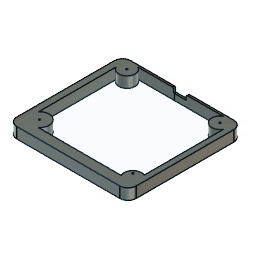
case (Autodesk Fusion 360 design; units mm, degrees)
description: KiCad electronic assembly
part number: case 1
Autodesk Fusion 360 part; units mm, degrees
(part 1 of 2)
sketch "Sketch1" plane through (0, 0, -0.05) normal (0, 0, -1) x (1, 0, 0)
  arc A0 (115.9024, 71.5818) -> (120.6818, 66.8024) centre (120.9, 71.8) ccw
  line L0 (120.6818, 66.8024) -> (120.9, 66.8)
  line L1 (120.9, 66.8) -> (209.95, 66.8)
  line L2 (209.95, 66.8) -> (210.1682, 66.8024)
  arc A1 (210.1682, 66.8024) -> (214.9476, 71.5818) centre (209.95, 71.8) ccw
  line L3 (214.9476, 71.5818) -> (214.95, 71.8)
  line L4 (214.95, 71.8) -> (214.95, 155.9)
  line L5 (214.95, 155.9) -> (214.9476, 156.1182)
  arc A2 (214.9476, 156.1182) -> (210.1682, 160.8976) centre (209.95, 155.9) ccw
  line L6 (210.1682, 160.8976) -> (209.95, 160.9)
  line L7 (209.95, 160.9) -> (120.9, 160.9)
  line L8 (120.9, 160.9) -> (120.6818, 160.8976)
  arc A3 (120.6818, 160.8976) -> (115.9024, 156.1182) centre (120.9, 155.9) ccw
  line L9 (115.9024, 156.1182) -> (115.9, 155.9)
  line L10 (115.9, 155.9) -> (115.9, 71.8)
  line L11 (115.9, 71.8) -> (115.9024, 71.5818)
  circle A4 centre (122.55, 154.05) radius 2.2
  circle A5 centre (208.4, 153.95) radius 2.2
  arc A6 (188.315, 150.698) -> (188.417, 150.8) centre (188.315, 150.8) ccw
  line L12 (188.315, 150.698) -> (187.415, 150.698)
  arc A7 (187.313, 150.8) -> (187.415, 150.698) centre (187.415, 150.8) ccw
  line L13 (187.313, 150.8) -> (187.313, 152.3)
  arc A8 (187.415, 152.402) -> (187.313, 152.3) centre (187.415, 152.3) ccw
  line L14 (187.415, 152.402) -> (188.315, 152.402)
  arc A9 (188.417, 152.3) -> (188.315, 152.402) centre (188.315, 152.3) ccw
  line L15 (188.417, 152.3) -> (188.417, 150.8)
  arc A10 (189.585, 150.698) -> (189.687, 150.8) centre (189.585, 150.8) ccw
  line L16 (189.585, 150.698) -> (188.685, 150.698)
  arc A11 (188.583, 150.8) -> (188.685, 150.698) centre (188.685, 150.8) ccw
  line L17 (188.583, 150.8) -> (188.583, 152.3)
  arc A12 (188.685, 152.402) -> (188.583, 152.3) centre (188.685, 152.3) ccw
  line L18 (188.685, 152.402) -> (189.585, 152.402)
  arc A13 (189.687, 152.3) -> (189.585, 152.402) centre (189.585, 152.3) ccw
  line L19 (189.687, 152.3) -> (189.687, 150.8)
  arc A14 (190.855, 150.698) -> (190.957, 150.8) centre (190.855, 150.8) ccw
  line L20 (190.855, 150.698) -> (189.955, 150.698)
  arc A15 (189.853, 150.8) -> (189.955, 150.698) centre (189.955, 150.8) ccw
  line L21 (189.853, 150.8) -> (189.853, 152.3)
  arc A16 (189.955, 152.402) -> (189.853, 152.3) centre (189.955, 152.3) ccw
  line L22 (189.955, 152.402) -> (190.855, 152.402)
  arc A17 (190.957, 152.3) -> (190.855, 152.402) centre (190.855, 152.3) ccw
  line L23 (190.957, 152.3) -> (190.957, 150.8)
  arc A18 (192.125, 150.698) -> (192.227, 150.8) centre (192.125, 150.8) ccw
  line L24 (192.125, 150.698) -> (191.225, 150.698)
  arc A19 (191.123, 150.8) -> (191.225, 150.698) centre (191.225, 150.8) ccw
  line L25 (191.123, 150.8) -> (191.123, 152.3)
  arc A20 (191.225, 152.402) -> (191.123, 152.3) centre (191.225, 152.3) ccw
  line L26 (191.225, 152.402) -> (192.125, 152.402)
  arc A21 (192.227, 152.3) -> (192.125, 152.402) centre (192.125, 152.3) ccw
  line L27 (192.227, 152.3) -> (192.227, 150.8)
  arc A22 (193.395, 150.698) -> (193.497, 150.8) centre (193.395, 150.8) ccw
  line L28 (193.395, 150.698) -> (192.495, 150.698)
  arc A23 (192.393, 150.8) -> (192.495, 150.698) centre (192.495, 150.8) ccw
  line L29 (192.393, 150.8) -> (192.393, 152.3)
  arc A24 (192.495, 152.402) -> (192.393, 152.3) centre (192.495, 152.3) ccw
  line L30 (192.495, 152.402) -> (193.395, 152.402)
  arc A25 (193.497, 152.3) -> (193.395, 152.402) centre (193.395, 152.3) ccw
  line L31 (193.497, 152.3) -> (193.497, 150.8)
  arc A26 (194.665, 150.698) -> (194.767, 150.8) centre (194.665, 150.8) ccw
  line L32 (194.665, 150.698) -> (193.765, 150.698)
  arc A27 (193.663, 150.8) -> (193.765, 150.698) centre (193.765, 150.8) ccw
  line L33 (193.663, 150.8) -> (193.663, 152.3)
  arc A28 (193.765, 152.402) -> (193.663, 152.3) centre (193.765, 152.3) ccw
  line L34 (193.765, 152.402) -> (194.665, 152.402)
  arc A29 (194.767, 152.3) -> (194.665, 152.402) centre (194.665, 152.3) ccw
  line L35 (194.767, 152.3) -> (194.767, 150.8)
  arc A30 (195.935, 150.698) -> (196.037, 150.8) centre (195.935, 150.8) ccw
  line L36 (195.935, 150.698) -> (195.035, 150.698)
  arc A31 (194.933, 150.8) -> (195.035, 150.698) centre (195.035, 150.8) ccw
  line L37 (194.933, 150.8) -> (194.933, 152.3)
  arc A32 (195.035, 152.402) -> (194.933, 152.3) centre (195.035, 152.3) ccw
  line L38 (195.035, 152.402) -> (195.935, 152.402)
  arc A33 (196.037, 152.3) -> (195.935, 152.402) centre (195.935, 152.3) ccw
  line L39 (196.037, 152.3) -> (196.037, 150.8)
  arc A34 (197.205, 150.698) -> (197.307, 150.8) centre (197.205, 150.8) ccw
  line L40 (197.205, 150.698) -> (196.305, 150.698)
  arc A35 (196.203, 150.8) -> (196.305, 150.698) centre (196.305, 150.8) ccw
  line L41 (196.203, 150.8) -> (196.203, 152.3)
  arc A36 (196.305, 152.402) -> (196.203, 152.3) centre (196.305, 152.3) ccw
  line L42 (196.305, 152.402) -> (197.205, 152.402)
  arc A37 (197.307, 152.3) -> (197.205, 152.402) centre (197.205, 152.3) ccw
  line L43 (197.307, 152.3) -> (197.307, 150.8)
  arc A38 (198.475, 150.698) -> (198.577, 150.8) centre (198.475, 150.8) ccw
  line L44 (198.475, 150.698) -> (197.575, 150.698)
  arc A39 (197.473, 150.8) -> (197.575, 150.698) centre (197.575, 150.8) ccw
  line L45 (197.473, 150.8) -> (197.473, 152.3)
  arc A40 (197.575, 152.402) -> (197.473, 152.3) centre (197.575, 152.3) ccw
  line L46 (197.575, 152.402) -> (198.475, 152.402)
  arc A41 (198.577, 152.3) -> (198.475, 152.402) centre (198.475, 152.3) ccw
  line L47 (198.577, 152.3) -> (198.577, 150.8)
  arc A42 (199.745, 150.698) -> (199.847, 150.8) centre (199.745, 150.8) ccw
  line L48 (199.745, 150.698) -> (198.845, 150.698)
  arc A43 (198.743, 150.8) -> (198.845, 150.698) centre (198.845, 150.8) ccw
  line L49 (198.743, 150.8) -> (198.743, 152.3)
  arc A44 (198.845, 152.402) -> (198.743, 152.3) centre (198.845, 152.3) ccw
  line L50 (198.845, 152.402) -> (199.745, 152.402)
  arc A45 (199.847, 152.3) -> (199.745, 152.402) centre (199.745, 152.3) ccw
  line L51 (199.847, 152.3) -> (199.847, 150.8)
  arc A46 (201.015, 150.698) -> (201.117, 150.8) centre (201.015, 150.8) ccw
  line L52 (201.015, 150.698) -> (200.115, 150.698)
  arc A47 (200.013, 150.8) -> (200.115, 150.698) centre (200.115, 150.8) ccw
  line L53 (200.013, 150.8) -> (200.013, 152.3)
  arc A48 (200.115, 152.402) -> (200.013, 152.3) centre (200.115, 152.3) ccw
  line L54 (200.115, 152.402) -> (201.015, 152.402)
  arc A49 (201.117, 152.3) -> (201.015, 152.402) centre (201.015, 152.3) ccw
  line L55 (201.117, 152.3) -> (201.117, 150.8)
  arc A50 (202.285, 150.698) -> (202.387, 150.8) centre (202.285, 150.8) ccw
  line L56 (202.285, 150.698) -> (201.385, 150.698)
  arc A51 (201.283, 150.8) -> (201.385, 150.698) centre (201.385, 150.8) ccw
  line L57 (201.283, 150.8) -> (201.283, 152.3)
  arc A52 (201.385, 152.402) -> (201.283, 152.3) centre (201.385, 152.3) ccw
  line L58 (201.385, 152.402) -> (202.285, 152.402)
  arc A53 (202.387, 152.3) -> (202.285, 152.402) centre (202.285, 152.3) ccw
  line L59 (202.387, 152.3) -> (202.387, 150.8)
  arc A54 (183.55, 150.523) -> (183.652, 150.625) centre (183.55, 150.625) ccw
  line L60 (183.55, 150.523) -> (181.4, 150.523)
  arc A55 (181.298, 150.625) -> (181.4, 150.523) centre (181.4, 150.625) ccw
  line L61 (181.298, 150.625) -> (181.298, 151.575)
  arc A56 (181.4, 151.677) -> (181.298, 151.575) centre (181.4, 151.575) ccw
  line L62 (181.4, 151.677) -> (183.55, 151.677)
  arc A57 (183.652, 151.575) -> (183.55, 151.677) centre (183.55, 151.575) ccw
  line L63 (183.652, 151.575) -> (183.652, 150.625)
  arc A58 (186.85, 149.748) -> (186.952, 149.85) centre (186.85, 149.85) ccw
  line L64 (186.85, 149.748) -> (185.35, 149.748)
  arc A59 (185.248, 149.85) -> (185.35, 149.748) centre (185.35, 149.85) ccw
  line L65 (185.248, 149.85) -> (185.248, 150.75)
  arc A60 (185.35, 150.852) -> (185.248, 150.75) centre (185.35, 150.75) ccw
  line L66 (185.35, 150.852) -> (186.85, 150.852)
  arc A61 (186.952, 150.75) -> (186.85, 150.852) centre (186.85, 150.75) ccw
  line L67 (186.952, 150.75) -> (186.952, 149.85)
  arc A62 (204.35, 149.748) -> (204.452, 149.85) centre (204.35, 149.85) ccw
  line L68 (204.35, 149.748) -> (202.85, 149.748)
  arc A63 (202.748, 149.85) -> (202.85, 149.748) centre (202.85, 149.85) ccw
  line L69 (202.748, 149.85) -> (202.748, 150.75)
  arc A64 (202.85, 150.852) -> (202.748, 150.75) centre (202.85, 150.75) ccw
  line L70 (202.85, 150.852) -> (204.35, 150.852)
  arc A65 (204.452, 150.75) -> (204.35, 150.852) centre (204.35, 150.75) ccw
  line L71 (204.452, 150.75) -> (204.452, 149.85)
  arc A66 (177.75, 147.073) -> (177.852, 147.175) centre (177.75, 147.175) ccw
  line L72 (177.75, 147.073) -> (175.6, 147.073)
  arc A67 (175.498, 147.175) -> (175.6, 147.073) centre (175.6, 147.175) ccw
  line L73 (175.498, 147.175) -> (175.498, 150.425)
  arc A68 (175.6, 150.527) -> (175.498, 150.425) centre (175.6, 150.425) ccw
  line L74 (175.6, 150.527) -> (177.75, 150.527)
  arc A69 (177.852, 150.425) -> (177.75, 150.527) centre (177.75, 150.425) ccw
  line L75 (177.852, 150.425) -> (177.852, 147.175)
  arc A70 (186.85, 148.478) -> (186.952, 148.58) centre (186.85, 148.58) ccw
  line L76 (186.85, 148.478) -> (185.35, 148.478)
  arc A71 (185.248, 148.58) -> (185.35, 148.478) centre (185.35, 148.58) ccw
  line L77 (185.248, 148.58) -> (185.248, 149.48)
  arc A72 (185.35, 149.582) -> (185.248, 149.48) centre (185.35, 149.48) ccw
  line L78 (185.35, 149.582) -> (186.85, 149.582)
  arc A73 (186.952, 149.48) -> (186.85, 149.582) centre (186.85, 149.48) ccw
  line L79 (186.952, 149.48) -> (186.952, 148.58)
  arc A74 (204.35, 148.478) -> (204.452, 148.58) centre (204.35, 148.58) ccw
  line L80 (204.35, 148.478) -> (202.85, 148.478)
  arc A75 (202.748, 148.58) -> (202.85, 148.478) centre (202.85, 148.58) ccw
  line L81 (202.748, 148.58) -> (202.748, 149.48)
  arc A76 (202.85, 149.582) -> (202.748, 149.48) centre (202.85, 149.48) ccw
  line L82 (202.85, 149.582) -> (204.35, 149.582)
  arc A77 (204.452, 149.48) -> (204.35, 149.582) centre (204.35, 149.48) ccw
  line L83 (204.452, 149.48) -> (204.452, 148.58)
  arc A78 (183.55, 148.223) -> (183.652, 148.325) centre (183.55, 148.325) ccw
  line L84 (183.55, 148.223) -> (181.4, 148.223)
  arc A79 (181.298, 148.325) -> (181.4, 148.223) centre (181.4, 148.325) ccw
  line L85 (181.298, 148.325) -> (181.298, 149.275)
  arc A80 (181.4, 149.377) -> (181.298, 149.275) centre (181.4, 149.275) ccw
  line L86 (181.4, 149.377) -> (183.55, 149.377)
  arc A81 (183.652, 149.275) -> (183.55, 149.377) centre (183.55, 149.275) ccw
  line L87 (183.652, 149.275) -> (183.652, 148.325)
  arc A82 (186.85, 147.208) -> (186.952, 147.31) centre (186.85, 147.31) ccw
  line L88 (186.85, 147.208) -> (185.35, 147.208)
  arc A83 (185.248, 147.31) -> (185.35, 147.208) centre (185.35, 147.31) ccw
  line L89 (185.248, 147.31) -> (185.248, 148.21)
  arc A84 (185.35, 148.312) -> (185.248, 148.21) centre (185.35, 148.21) ccw
  line L90 (185.35, 148.312) -> (186.85, 148.312)
  arc A85 (186.952, 148.21) -> (186.85, 148.312) centre (186.85, 148.21) ccw
  line L91 (186.952, 148.21) -> (186.952, 147.31)
  arc A86 (204.35, 147.208) -> (204.452, 147.31) centre (204.35, 147.31) ccw
  line L92 (204.35, 147.208) -> (202.85, 147.208)
  arc A87 (202.748, 147.31) -> (202.85, 147.208) centre (202.85, 147.31) ccw
  line L93 (202.748, 147.31) -> (202.748, 148.21)
  arc A88 (202.85, 148.312) -> (202.748, 148.21) centre (202.85, 148.21) ccw
  line L94 (202.85, 148.312) -> (204.35, 148.312)
  arc A89 (204.452, 148.21) -> (204.35, 148.312) centre (204.35, 148.21) ccw
  line L95 (204.452, 148.21) -> (204.452, 147.31)
  arc A90 (183.55, 145.923) -> (183.652, 146.025) centre (183.55, 146.025) ccw
  line L96 (183.55, 145.923) -> (181.4, 145.923)
  arc A91 (181.298, 146.025) -> (181.4, 145.923) centre (181.4, 146.025) ccw
  line L97 (181.298, 146.025) -> (181.298, 146.975)
  arc A92 (181.4, 147.077) -> (181.298, 146.975) centre (181.4, 146.975) ccw
  line L98 (181.4, 147.077) -> (183.55, 147.077)
  arc A93 (183.652, 146.975) -> (183.55, 147.077) centre (183.55, 146.975) ccw
  line L99 (183.652, 146.975) -> (183.652, 146.025)
  arc A94 (186.85, 145.938) -> (186.952, 146.04) centre (186.85, 146.04) ccw
  line L100 (186.85, 145.938) -> (185.35, 145.938)
  arc A95 (185.248, 146.04) -> (185.35, 145.938) centre (185.35, 146.04) ccw
  line L101 (185.248, 146.04) -> (185.248, 146.94)
  arc A96 (185.35, 147.042) -> (185.248, 146.94) centre (185.35, 146.94) ccw
  line L102 (185.35, 147.042) -> (186.85, 147.042)
  arc A97 (186.952, 146.94) -> (186.85, 147.042) centre (186.85, 146.94) ccw
  line L103 (186.952, 146.94) -> (186.952, 146.04)
  arc A98 (204.35, 145.938) -> (204.452, 146.04) centre (204.35, 146.04) ccw
  line L104 (204.35, 145.938) -> (202.85, 145.938)
  arc A99 (202.748, 146.04) -> (202.85, 145.938) centre (202.85, 146.04) ccw
  line L105 (202.748, 146.04) -> (202.748, 146.94)
  arc A100 (202.85, 147.042) -> (202.748, 146.94) centre (202.85, 146.94) ccw
  line L106 (202.85, 147.042) -> (204.35, 147.042)
  arc A101 (204.452, 146.94) -> (204.35, 147.042) centre (204.35, 146.94) ccw
  line L107 (204.452, 146.94) -> (204.452, 146.04)
  arc A102 (186.85, 144.668) -> (186.952, 144.77) centre (186.85, 144.77) ccw
  line L108 (186.85, 144.668) -> (185.35, 144.668)
  arc A103 (185.248, 144.77) -> (185.35, 144.668) centre (185.35, 144.77) ccw
  line L109 (185.248, 144.77) -> (185.248, 145.67)
  arc A104 (185.35, 145.772) -> (185.248, 145.67) centre (185.35, 145.67) ccw
  line L110 (185.35, 145.772) -> (186.85, 145.772)
  arc A105 (186.952, 145.67) -> (186.85, 145.772) centre (186.85, 145.67) ccw
  line L111 (186.952, 145.67) -> (186.952, 144.77)
  arc A106 (204.35, 144.668) -> (204.452, 144.77) centre (204.35, 144.77) ccw
  line L112 (204.35, 144.668) -> (202.85, 144.668)
  arc A107 (202.748, 144.77) -> (202.85, 144.668) centre (202.85, 144.77) ccw
  line L113 (202.748, 144.77) -> (202.748, 145.67)
  arc A108 (202.85, 145.772) -> (202.748, 145.67) centre (202.85, 145.67) ccw
  line L114 (202.85, 145.772) -> (204.35, 145.772)
  arc A109 (204.452, 145.67) -> (204.35, 145.772) centre (204.35, 145.67) ccw
  line L115 (204.452, 145.67) -> (204.452, 144.77)
  circle A110 centre (165.24, 143.58) radius 2
  arc A111 (186.85, 143.398) -> (186.952, 143.5) centre (186.85, 143.5) ccw
  line L116 (186.85, 143.398) -> (185.35, 143.398)
  arc A112 (185.248, 143.5) -> (185.35, 143.398) centre (185.35, 143.5) ccw
  line L117 (185.248, 143.5) -> (185.248, 144.4)
  arc A113 (185.35, 144.502) -> (185.248, 144.4) centre (185.35, 144.4) ccw
  line L118 (185.35, 144.502) -> (186.85, 144.502)
  arc A114 (186.952, 144.4) -> (186.85, 144.502) centre (186.85, 144.4) ccw
  line L119 (186.952, 144.4) -> (186.952, 143.5)
  arc A115 (204.35, 143.398) -> (204.452, 143.5) centre (204.35, 143.5) ccw
  line L120 (204.35, 143.398) -> (202.85, 143.398)
  arc A116 (202.748, 143.5) -> (202.85, 143.398) centre (202.85, 143.5) ccw
  line L121 (202.748, 143.5) -> (202.748, 144.4)
  arc A117 (202.85, 144.502) -> (202.748, 144.4) centre (202.85, 144.4) ccw
  line L122 (202.85, 144.502) -> (204.35, 144.502)
  arc A118 (204.452, 144.4) -> (204.35, 144.502) centre (204.35, 144.4) ccw
  line L123 (204.452, 144.4) -> (204.452, 143.5)
  circle A119 centre (160.16, 143.58) radius 0.85
  circle A120 centre (170.32, 143.58) radius 0.85
  arc A121 (178.525, 143.2) -> (178.775, 143.45) centre (178.525, 143.45) ccw
  line L124 (178.525, 143.2) -> (177.575, 143.2)
  arc A122 (177.325, 143.45) -> (177.575, 143.2) centre (177.575, 143.45) ccw
  line L125 (177.325, 143.45) -> (177.325, 143.95)
  arc A123 (177.575, 144.2) -> (177.325, 143.95) centre (177.575, 143.95) ccw
  line L126 (177.575, 144.2) -> (178.525, 144.2)
  arc A124 (178.775, 143.95) -> (178.525, 144.2) centre (178.525, 143.95) ccw
  line L127 (178.775, 143.95) -> (178.775, 143.45)
  arc A125 (195.4, 142.358) -> (195.502, 142.46) centre (195.4, 142.46) ccw
  line L128 (195.4, 142.358) -> (194.5, 142.358)
  arc A126 (194.398, 142.46) -> (194.5, 142.358) centre (194.5, 142.46) ccw
  line L129 (194.398, 142.46) -> (194.398, 143.36)
  arc A127 (194.5, 143.462) -> (194.398, 143.36) centre (194.5, 143.36) ccw
  line L130 (194.5, 143.462) -> (195.4, 143.462)
  arc A128 (195.502, 143.36) -> (195.4, 143.462) centre (195.4, 143.36) ccw
  line L131 (195.502, 143.36) -> (195.502, 142.46)
  arc A129 (196.8, 142.358) -> (196.902, 142.46) centre (196.8, 142.46) ccw
  line L132 (196.8, 142.358) -> (195.9, 142.358)
  arc A130 (195.798, 142.46) -> (195.9, 142.358) centre (195.9, 142.46) ccw
  line L133 (195.798, 142.46) -> (195.798, 143.36)
  arc A131 (195.9, 143.462) -> (195.798, 143.36) centre (195.9, 143.36) ccw
  line L134 (195.9, 143.462) -> (196.8, 143.462)
  arc A132 (196.902, 143.36) -> (196.8, 143.462) centre (196.8, 143.36) ccw
  line L135 (196.902, 143.36) -> (196.902, 142.46)
  arc A133 (198.2, 142.358) -> (198.302, 142.46) centre (198.2, 142.46) ccw
  line L136 (198.2, 142.358) -> (197.3, 142.358)
  arc A134 (197.198, 142.46) -> (197.3, 142.358) centre (197.3, 142.46) ccw
  line L137 (197.198, 142.46) -> (197.198, 143.36)
  arc A135 (197.3, 143.462) -> (197.198, 143.36) centre (197.3, 143.36) ccw
  line L138 (197.3, 143.462) -> (198.2, 143.462)
  arc A136 (198.302, 143.36) -> (198.2, 143.462) centre (198.2, 143.36) ccw
  line L139 (198.302, 143.36) -> (198.302, 142.46)
  arc A137 (186.85, 142.128) -> (186.952, 142.23) centre (186.85, 142.23) ccw
  line L140 (186.85, 142.128) -> (185.35, 142.128)
  arc A138 (185.248, 142.23) -> (185.35, 142.128) centre (185.35, 142.23) ccw
  line L141 (185.248, 142.23) -> (185.248, 143.13)
  arc A139 (185.35, 143.232) -> (185.248, 143.13) centre (185.35, 143.13) ccw
  line L142 (185.35, 143.232) -> (186.85, 143.232)
  arc A140 (186.952, 143.13) -> (186.85, 143.232) centre (186.85, 143.13) ccw
  line L143 (186.952, 143.13) -> (186.952, 142.23)
  arc A141 (204.35, 142.128) -> (204.452, 142.23) centre (204.35, 142.23) ccw
  line L144 (204.35, 142.128) -> (202.85, 142.128)
  arc A142 (202.748, 142.23) -> (202.85, 142.128) centre (202.85, 142.23) ccw
  line L145 (202.748, 142.23) -> (202.748, 143.13)
  arc A143 (202.85, 143.232) -> (202.748, 143.13) centre (202.85, 143.13) ccw
  line L146 (202.85, 143.232) -> (204.35, 143.232)
  arc A144 (204.452, 143.13) -> (204.35, 143.232) centre (204.35, 143.13) ccw
  line L147 (204.452, 143.13) -> (204.452, 142.23)
  arc A145 (178.525, 141.3) -> (178.775, 141.55) centre (178.525, 141.55) ccw
  line L148 (178.525, 141.3) -> (177.575, 141.3)
  arc A146 (177.325, 141.55) -> (177.575, 141.3) centre (177.575, 141.55) ccw
  line L149 (177.325, 141.55) -> (177.325, 142.05)
  arc A147 (177.575, 142.3) -> (177.325, 142.05) centre (177.575, 142.05) ccw
  line L150 (177.575, 142.3) -> (178.525, 142.3)
  arc A148 (178.775, 142.05) -> (178.525, 142.3) centre (178.525, 142.05) ccw
  line L151 (178.775, 142.05) -> (178.775, 141.55)
  circle A149 centre (161.43, 141.04) radius 1.1
  arc A150 (195.4, 140.958) -> (195.502, 141.06) centre (195.4, 141.06) ccw
  line L152 (195.4, 140.958) -> (194.5, 140.958)
  arc A151 (194.398, 141.06) -> (194.5, 140.958) centre (194.5, 141.06) ccw
  line L153 (194.398, 141.06) -> (194.398, 141.96)
  arc A152 (194.5, 142.062) -> (194.398, 141.96) centre (194.5, 141.96) ccw
  line L154 (194.5, 142.062) -> (195.4, 142.062)
  arc A153 (195.502, 141.96) -> (195.4, 142.062) centre (195.4, 141.96) ccw
  line L155 (195.502, 141.96) -> (195.502, 141.06)
  arc A154 (196.8, 140.958) -> (196.902, 141.06) centre (196.8, 141.06) ccw
  line L156 (196.8, 140.958) -> (195.9, 140.958)
  arc A155 (195.798, 141.06) -> (195.9, 140.958) centre (195.9, 141.06) ccw
  line L157 (195.798, 141.06) -> (195.798, 141.96)
  arc A156 (195.9, 142.062) -> (195.798, 141.96) centre (195.9, 141.96) ccw
  line L158 (195.9, 142.062) -> (196.8, 142.062)
  arc A157 (196.902, 141.96) -> (196.8, 142.062) centre (196.8, 141.96) ccw
  line L159 (196.902, 141.96) -> (196.902, 141.06)
  arc A158 (198.2, 140.958) -> (198.302, 141.06) centre (198.2, 141.06) ccw
  line L160 (198.2, 140.958) -> (197.3, 140.958)
  arc A159 (197.198, 141.06) -> (197.3, 140.958) centre (197.3, 141.06) ccw
  line L161 (197.198, 141.06) -> (197.198, 141.96)
  arc A160 (197.3, 142.062) -> (197.198, 141.96) centre (197.3, 141.96) ccw
  line L162 (197.3, 142.062) -> (198.2, 142.062)
  arc A161 (198.302, 141.96) -> (198.2, 142.062) centre (198.2, 141.96) ccw
  line L163 (198.302, 141.96) -> (198.302, 141.06)
  arc A162 (186.85, 140.858) -> (186.952, 140.96) centre (186.85, 140.96) ccw
  line L164 (186.85, 140.858) -> (185.35, 140.858)
  arc A163 (185.248, 140.96) -> (185.35, 140.858) centre (185.35, 140.96) ccw
  line L165 (185.248, 140.96) -> (185.248, 141.86)
  arc A164 (185.35, 141.962) -> (185.248, 141.86) centre (185.35, 141.86) ccw
  line L166 (185.35, 141.962) -> (186.85, 141.962)
  arc A165 (186.952, 141.86) -> (186.85, 141.962) centre (186.85, 141.86) ccw
  line L167 (186.952, 141.86) -> (186.952, 140.96)
  arc A166 (204.35, 140.858) -> (204.452, 140.96) centre (204.35, 140.96) ccw
  line L168 (204.35, 140.858) -> (202.85, 140.858)
  arc A167 (202.748, 140.96) -> (202.85, 140.858) centre (202.85, 140.96) ccw
  line L169 (202.748, 140.96) -> (202.748, 141.86)
  arc A168 (202.85, 141.962) -> (202.748, 141.86) centre (202.85, 141.86) ccw
  line L170 (202.85, 141.962) -> (204.35, 141.962)
  arc A169 (204.452, 141.86) -> (204.35, 141.962) centre (204.35, 141.86) ccw
  line L171 (204.452, 141.86) -> (204.452, 140.96)
  arc A170 (186.85, 139.588) -> (186.952, 139.69) centre (186.85, 139.69) ccw
  line L172 (186.85, 139.588) -> (185.35, 139.588)
  arc A171 (185.248, 139.69) -> (185.35, 139.588) centre (185.35, 139.69) ccw
  line L173 (185.248, 139.69) -> (185.248, 140.59)
  arc A172 (185.35, 140.692) -> (185.248, 140.59) centre (185.35, 140.59) ccw
  line L174 (185.35, 140.692) -> (186.85, 140.692)
  arc A173 (186.952, 140.59) -> (186.85, 140.692) centre (186.85, 140.59) ccw
  line L175 (186.952, 140.59) -> (186.952, 139.69)
  arc A174 (204.35, 139.588) -> (204.452, 139.69) centre (204.35, 139.69) ccw
  line L176 (204.35, 139.588) -> (202.85, 139.588)
  arc A175 (202.748, 139.69) -> (202.85, 139.588) centre (202.85, 139.69) ccw
  line L177 (202.748, 139.69) -> (202.748, 140.59)
  arc A176 (202.85, 140.692) -> (202.748, 140.59) centre (202.85, 140.59) ccw
  line L178 (202.85, 140.692) -> (204.35, 140.692)
  arc A177 (204.452, 140.59) -> (204.35, 140.692) centre (204.35, 140.59) ccw
  line L179 (204.452, 140.59) -> (204.452, 139.69)
  arc A178 (195.4, 139.558) -> (195.502, 139.66) centre (195.4, 139.66) ccw
  line L180 (195.4, 139.558) -> (194.5, 139.558)
  arc A179 (194.398, 139.66) -> (194.5, 139.558) centre (194.5, 139.66) ccw
  line L181 (194.398, 139.66) -> (194.398, 140.56)
  arc A180 (194.5, 140.662) -> (194.398, 140.56) centre (194.5, 140.56) ccw
  line L182 (194.5, 140.662) -> (195.4, 140.662)
  arc A181 (195.502, 140.56) -> (195.4, 140.662) centre (195.4, 140.56) ccw
  line L183 (195.502, 140.56) -> (195.502, 139.66)
  arc A182 (196.8, 139.558) -> (196.902, 139.66) centre (196.8, 139.66) ccw
  line L184 (196.8, 139.558) -> (195.9, 139.558)
  arc A183 (195.798, 139.66) -> (195.9, 139.558) centre (195.9, 139.66) ccw
  line L185 (195.798, 139.66) -> (195.798, 140.56)
  arc A184 (195.9, 140.662) -> (195.798, 140.56) centre (195.9, 140.56) ccw
  line L186 (195.9, 140.662) -> (196.8, 140.662)
  arc A185 (196.902, 140.56) -> (196.8, 140.662) centre (196.8, 140.56) ccw
  line L187 (196.902, 140.56) -> (196.902, 139.66)
  arc A186 (198.2, 139.558) -> (198.302, 139.66) centre (198.2, 139.66) ccw
  line L188 (198.2, 139.558) -> (197.3, 139.558)
  arc A187 (197.198, 139.66) -> (197.3, 139.558) centre (197.3, 139.66) ccw
  line L189 (197.198, 139.66) -> (197.198, 140.56)
  arc A188 (197.3, 140.662) -> (197.198, 140.56) centre (197.3, 140.56) ccw
  line L190 (197.3, 140.662) -> (198.2, 140.662)
  arc A189 (198.302, 140.56) -> (198.2, 140.662) centre (198.2, 140.56) ccw
  line L191 (198.302, 140.56) -> (198.302, 139.66)
  circle A190 centre (167.78, 138.5) radius 1.1
  arc A191 (186.85, 138.318) -> (186.952, 138.42) centre (186.85, 138.42) ccw
  line L192 (186.85, 138.318) -> (185.35, 138.318)
  arc A192 (185.248, 138.42) -> (185.35, 138.318) centre (185.35, 138.42) ccw
  line L193 (185.248, 138.42) -> (185.248, 139.32)
  arc A193 (185.35, 139.422) -> (185.248, 139.32) centre (185.35, 139.32) ccw
  line L194 (185.35, 139.422) -> (186.85, 139.422)
  arc A194 (186.952, 139.32) -> (186.85, 139.422) centre (186.85, 139.32) ccw
  line L195 (186.952, 139.32) -> (186.952, 138.42)
  arc A195 (204.35, 138.318) -> (204.452, 138.42) centre (204.35, 138.42) ccw
  line L196 (204.35, 138.318) -> (202.85, 138.318)
  arc A196 (202.748, 138.42) -> (202.85, 138.318) centre (202.85, 138.42) ccw
  line L197 (202.748, 138.42) -> (202.748, 139.32)
  arc A197 (202.85, 139.422) -> (202.748, 139.32) centre (202.85, 139.32) ccw
  line L198 (202.85, 139.422) -> (204.35, 139.422)
  arc A198 (204.452, 139.32) -> (204.35, 139.422) centre (204.35, 139.32) ccw
  line L199 (204.452, 139.32) -> (204.452, 138.42)
  arc A199 (132.5, 137.7) -> (132.75, 137.95) centre (132.5, 137.95) ccw
  line L200 (132.5, 137.7) -> (131.6, 137.7)
  arc A200 (131.35, 137.95) -> (131.6, 137.7) centre (131.6, 137.95) ccw
  line L201 (131.35, 137.95) -> (131.35, 138.475)
  arc A201 (131.6, 138.725) -> (131.35, 138.475) centre (131.6, 138.475) ccw
  line L202 (131.6, 138.725) -> (132.5, 138.725)
  arc A202 (132.75, 138.475) -> (132.5, 138.725) centre (132.5, 138.475) ccw
  line L203 (132.75, 138.475) -> (132.75, 137.95)
  arc A203 (137.8, 137.55) -> (138.05, 137.8) centre (137.8, 137.8) ccw
  line L204 (137.8, 137.55) -> (136.9, 137.55)
  arc A204 (136.65, 137.8) -> (136.9, 137.55) centre (136.9, 137.8) ccw
  line L205 (136.65, 137.8) -> (136.65, 138.325)
  arc A205 (136.9, 138.575) -> (136.65, 138.325) centre (136.9, 138.325) ccw
  line L206 (136.9, 138.575) -> (137.8, 138.575)
  arc A206 (138.05, 138.325) -> (137.8, 138.575) centre (137.8, 138.325) ccw
  line L207 (138.05, 138.325) -> (138.05, 137.8)
  arc A207 (186.85, 137.048) -> (186.952, 137.15) centre (186.85, 137.15) ccw
  line L208 (186.85, 137.048) -> (185.35, 137.048)
  arc A208 (185.248, 137.15) -> (185.35, 137.048) centre (185.35, 137.15) ccw
  line L209 (185.248, 137.15) -> (185.248, 138.05)
  arc A209 (185.35, 138.152) -> (185.248, 138.05) centre (185.35, 138.05) ccw
  line L210 (185.35, 138.152) -> (186.85, 138.152)
  arc A210 (186.952, 138.05) -> (186.85, 138.152) centre (186.85, 138.05) ccw
  line L211 (186.952, 138.05) -> (186.952, 137.15)
  arc A211 (204.35, 137.048) -> (204.452, 137.15) centre (204.35, 137.15) ccw
  line L212 (204.35, 137.048) -> (202.85, 137.048)
  arc A212 (202.748, 137.15) -> (202.85, 137.048) centre (202.85, 137.15) ccw
  line L213 (202.748, 137.15) -> (202.748, 138.05)
  arc A213 (202.85, 138.152) -> (202.748, 138.05) centre (202.85, 138.05) ccw
  line L214 (202.85, 138.152) -> (204.35, 138.152)
  arc A214 (204.452, 138.05) -> (204.35, 138.152) centre (204.35, 138.05) ccw
  line L215 (204.452, 138.05) -> (204.452, 137.15)
  arc A215 (132.5, 135.875) -> (132.75, 136.125) centre (132.5, 136.125) ccw
  line L216 (132.5, 135.875) -> (131.6, 135.875)
  arc A216 (131.35, 136.125) -> (131.6, 135.875) centre (131.6, 136.125) ccw
  line L217 (131.35, 136.125) -> (131.35, 136.65)
  arc A217 (131.6, 136.9) -> (131.35, 136.65) centre (131.6, 136.65) ccw
  line L218 (131.6, 136.9) -> (132.5, 136.9)
  arc A218 (132.75, 136.65) -> (132.5, 136.9) centre (132.5, 136.65) ccw
  line L219 (132.75, 136.65) -> (132.75, 136.125)
  arc A219 (186.85, 135.778) -> (186.952, 135.88) centre (186.85, 135.88) ccw
  line L220 (186.85, 135.778) -> (185.35, 135.778)
  arc A220 (185.248, 135.88) -> (185.35, 135.778) centre (185.35, 135.88) ccw
  line L221 (185.248, 135.88) -> (185.248, 136.78)
  arc A221 (185.35, 136.882) -> (185.248, 136.78) centre (185.35, 136.78) ccw
  line L222 (185.35, 136.882) -> (186.85, 136.882)
  arc A222 (186.952, 136.78) -> (186.85, 136.882) centre (186.85, 136.78) ccw
  line L223 (186.952, 136.78) -> (186.952, 135.88)
  arc A223 (204.35, 135.778) -> (204.452, 135.88) centre (204.35, 135.88) ccw
  line L224 (204.35, 135.778) -> (202.85, 135.778)
  arc A224 (202.748, 135.88) -> (202.85, 135.778) centre (202.85, 135.88) ccw
  line L225 (202.748, 135.88) -> (202.748, 136.78)
  arc A225 (202.85, 136.882) -> (202.748, 136.78) centre (202.85, 136.78) ccw
  line L226 (202.85, 136.882) -> (204.35, 136.882)
  arc A226 (204.452, 136.78) -> (204.35, 136.882) centre (204.35, 136.78) ccw
  line L227 (204.452, 136.78) -> (204.452, 135.88)
  arc A227 (137.8, 135.725) -> (138.05, 135.975) centre (137.8, 135.975) ccw
  line L228 (137.8, 135.725) -> (136.9, 135.725)
  arc A228 (136.65, 135.975) -> (136.9, 135.725) centre (136.9, 135.975) ccw
  line L229 (136.65, 135.975) -> (136.65, 136.5)
  arc A229 (136.9, 136.75) -> (136.65, 136.5) centre (136.9, 136.5) ccw
  line L230 (136.9, 136.75) -> (137.8, 136.75)
  arc A230 (138.05, 136.5) -> (137.8, 136.75) centre (137.8, 136.5) ccw
  line L231 (138.05, 136.5) -> (138.05, 135.975)
  arc A231 (206.925, 135.6) -> (207.175, 135.85) centre (206.925, 135.85) ccw
  line L232 (206.925, 135.6) -> (205.975, 135.6)
  arc A232 (205.725, 135.85) -> (205.975, 135.6) centre (205.975, 135.85) ccw
  line L233 (205.725, 135.85) -> (205.725, 136.35)
  arc A233 (205.975, 136.6) -> (205.725, 136.35) centre (205.975, 136.35) ccw
  line L234 (205.975, 136.6) -> (206.925, 136.6)
  arc A234 (207.175, 136.35) -> (206.925, 136.6) centre (206.925, 136.35) ccw
  line L235 (207.175, 136.35) -> (207.175, 135.85)
  arc A235 (186.85, 134.508) -> (186.952, 134.61) centre (186.85, 134.61) ccw
  line L236 (186.85, 134.508) -> (185.35, 134.508)
  arc A236 (185.248, 134.61) -> (185.35, 134.508) centre (185.35, 134.61) ccw
  line L237 (185.248, 134.61) -> (185.248, 135.51)
  arc A237 (185.35, 135.612) -> (185.248, 135.51) centre (185.35, 135.51) ccw
  line L238 (185.35, 135.612) -> (186.85, 135.612)
  arc A238 (186.952, 135.51) -> (186.85, 135.612) centre (186.85, 135.51) ccw
  line L239 (186.952, 135.51) -> (186.952, 134.61)
  arc A239 (204.35, 134.508) -> (204.452, 134.61) centre (204.35, 134.61) ccw
  line L240 (204.35, 134.508) -> (202.85, 134.508)
  arc A240 (202.748, 134.61) -> (202.85, 134.508) centre (202.85, 134.61) ccw
  line L241 (202.748, 134.61) -> (202.748, 135.51)
  arc A241 (202.85, 135.612) -> (202.748, 135.51) centre (202.85, 135.51) ccw
  line L242 (202.85, 135.612) -> (204.35, 135.612)
  arc A242 (204.452, 135.51) -> (204.35, 135.612) centre (204.35, 135.51) ccw
  line L243 (204.452, 135.51) -> (204.452, 134.61)
  arc A243 (206.925, 133.7) -> (207.175, 133.95) centre (206.925, 133.95) ccw
  line L244 (206.925, 133.7) -> (205.975, 133.7)
  arc A244 (205.725, 133.95) -> (205.975, 133.7) centre (205.975, 133.95) ccw
  line L245 (205.725, 133.95) -> (205.725, 134.45)
  arc A245 (205.975, 134.7) -> (205.725, 134.45) centre (205.975, 134.45) ccw
  line L246 (205.975, 134.7) -> (206.925, 134.7)
  arc A246 (207.175, 134.45) -> (206.925, 134.7) centre (206.925, 134.45) ccw
  line L247 (207.175, 134.45) -> (207.175, 133.95)
  arc A247 (186.85, 133.238) -> (186.952, 133.34) centre (186.85, 133.34) ccw
  line L248 (186.85, 133.238) -> (185.35, 133.238)
  arc A248 (185.248, 133.34) -> (185.35, 133.238) centre (185.35, 133.34) ccw
  line L249 (185.248, 133.34) -> (185.248, 134.24)
  arc A249 (185.35, 134.342) -> (185.248, 134.24) centre (185.35, 134.24) ccw
  line L250 (185.35, 134.342) -> (186.85, 134.342)
  arc A250 (186.952, 134.24) -> (186.85, 134.342) centre (186.85, 134.24) ccw
  line L251 (186.952, 134.24) -> (186.952, 133.34)
  arc A251 (204.35, 133.238) -> (204.452, 133.34) centre (204.35, 133.34) ccw
  line L252 (204.35, 133.238) -> (202.85, 133.238)
  arc A252 (202.748, 133.34) -> (202.85, 133.238) centre (202.85, 133.34) ccw
  line L253 (202.748, 133.34) -> (202.748, 134.24)
  arc A253 (202.85, 134.342) -> (202.748, 134.24) centre (202.85, 134.24) ccw
  line L254 (202.85, 134.342) -> (204.35, 134.342)
  arc A254 (204.452, 134.24) -> (204.35, 134.342) centre (204.35, 134.24) ccw
  line L255 (204.452, 134.24) -> (204.452, 133.34)
  arc A255 (144.65, 132.95) -> (144.9, 133.2) centre (144.65, 133.2) ccw
  line L256 (144.65, 132.95) -> (143.75, 132.95)
  arc A256 (143.5, 133.2) -> (143.75, 132.95) centre (143.75, 133.2) ccw
  line L257 (143.5, 133.2) -> (143.5, 133.725)
  arc A257 (143.75, 133.975) -> (143.5, 133.725) centre (143.75, 133.725) ccw
  line L258 (143.75, 133.975) -> (144.65, 133.975)
  arc A258 (144.9, 133.725) -> (144.65, 133.975) centre (144.65, 133.725) ccw
  line L259 (144.9, 133.725) -> (144.9, 133.2)
  arc A259 (144.65, 131.125) -> (144.9, 131.375) centre (144.65, 131.375) ccw
  line L260 (144.65, 131.125) -> (143.75, 131.125)
  arc A260 (143.5, 131.375) -> (143.75, 131.125) centre (143.75, 131.375) ccw
  line L261 (143.5, 131.375) -> (143.5, 131.9)
  arc A261 (143.75, 132.15) -> (143.5, 131.9) centre (143.75, 131.9) ccw
  line L262 (143.75, 132.15) -> (144.65, 132.15)
  arc A262 (144.9, 131.9) -> (144.65, 132.15) centre (144.65, 131.9) ccw
  line L263 (144.9, 131.9) -> (144.9, 131.375)
  circle A263 centre (155.356, 124.5071) radius 2
  circle A264 centre (174.4162, 124.5068) radius 2
  circle A265 centre (150.276, 124.5071) radius 0.85
  circle A266 centre (160.436, 124.5071) radius 0.85
  circle A267 centre (169.3362, 124.5068) radius 0.85
  circle A268 centre (179.4962, 124.5068) radius 0.85
  circle A269 centre (151.546, 121.9671) radius 1.1
  circle A270 centre (170.6062, 121.9668) radius 1.1
  circle A271 centre (157.896, 119.4271) radius 1.1
  circle A272 centre (176.9562, 119.4268) radius 1.1
  circle A273 centre (193.5, 115.37) radius 2
  circle A274 centre (136.34, 114.88) radius 2
  circle A275 centre (188.42, 115.37) radius 0.85
  circle A276 centre (198.58, 115.37) radius 0.85
  circle A277 centre (131.26, 114.88) radius 0.85
  circle A278 centre (141.42, 114.88) radius 0.85
  circle A279 centre (189.69, 112.83) radius 1.1
  circle A280 centre (132.53, 112.34) radius 1.1
  circle A281 centre (196.04, 110.29) radius 1.1
  circle A282 centre (138.88, 109.8) radius 1.1
  arc A283 (206.725, 108.2) -> (206.975, 108.45) centre (206.725, 108.45) ccw
  line L264 (206.725, 108.2) -> (205.775, 108.2)
  arc A284 (205.525, 108.45) -> (205.775, 108.2) centre (205.775, 108.45) ccw
  line L265 (205.525, 108.45) -> (205.525, 108.95)
  arc A285 (205.775, 109.2) -> (205.525, 108.95) centre (205.775, 108.95) ccw
  line L266 (205.775, 109.2) -> (206.725, 109.2)
  arc A286 (206.975, 108.95) -> (206.725, 109.2) centre (206.725, 108.95) ccw
  line L267 (206.975, 108.95) -> (206.975, 108.45)
  circle A287 centre (155.36, 105.48) radius 2
  circle A288 centre (174.41, 105.48) radius 2
  arc A289 (206.725, 106.3) -> (206.975, 106.55) centre (206.725, 106.55) ccw
  line L268 (206.725, 106.3) -> (205.775, 106.3)
  arc A290 (205.525, 106.55) -> (205.775, 106.3) centre (205.775, 106.55) ccw
  line L269 (205.525, 106.55) -> (205.525, 107.05)
  arc A291 (205.775, 107.3) -> (205.525, 107.05) centre (205.775, 107.05) ccw
  line L270 (205.775, 107.3) -> (206.725, 107.3)
  arc A292 (206.975, 107.05) -> (206.725, 107.3) centre (206.725, 107.05) ccw
  line L271 (206.975, 107.05) -> (206.975, 106.55)
  circle A293 centre (150.28, 105.48) radius 0.85
  circle A294 centre (160.44, 105.48) radius 0.85
  circle A295 centre (169.33, 105.48) radius 0.85
  circle A296 centre (179.49, 105.48) radius 0.85
  arc A297 (206.75, 104.05) -> (207, 104.3) centre (206.75, 104.3) ccw
  line L272 (206.75, 104.05) -> (205.85, 104.05)
  arc A298 (205.6, 104.3) -> (205.85, 104.05) centre (205.85, 104.3) ccw
  line L273 (205.6, 104.3) -> (205.6, 104.825)
  arc A299 (205.85, 105.075) -> (205.6, 104.825) centre (205.85, 104.825) ccw
  line L274 (205.85, 105.075) -> (206.75, 105.075)
  arc A300 (207, 104.825) -> (206.75, 105.075) centre (206.75, 104.825) ccw
  line L275 (207, 104.825) -> (207, 104.3)
  circle A301 centre (151.55, 102.94) radius 1.1
  circle A302 centre (170.6, 102.94) radius 1.1
  arc A303 (206.75, 102.225) -> (207, 102.475) centre (206.75, 102.475) ccw
  line L276 (206.75, 102.225) -> (205.85, 102.225)
  arc A304 (205.6, 102.475) -> (205.85, 102.225) centre (205.85, 102.475) ccw
  line L277 (205.6, 102.475) -> (205.6, 103)
  arc A305 (205.85, 103.25) -> (205.6, 103) centre (205.85, 103) ccw
  line L278 (205.85, 103.25) -> (206.75, 103.25)
  arc A306 (207, 103) -> (206.75, 103.25) centre (206.75, 103) ccw
  line L279 (207, 103) -> (207, 102.475)
  arc A307 (186.85, 100.898) -> (186.952, 101) centre (186.85, 101) ccw
  line L280 (186.85, 100.898) -> (185.35, 100.898)
  arc A308 (185.248, 101) -> (185.35, 100.898) centre (185.35, 101) ccw
  line L281 (185.248, 101) -> (185.248, 102.4)
  arc A309 (185.35, 102.502) -> (185.248, 102.4) centre (185.35, 102.4) ccw
  line L282 (185.35, 102.502) -> (186.85, 102.502)
  arc A310 (186.952, 102.4) -> (186.85, 102.502) centre (186.85, 102.4) ccw
  line L283 (186.952, 102.4) -> (186.952, 101)
  arc A311 (193.35, 100.898) -> (193.452, 101) centre (193.35, 101) ccw
  line L284 (193.35, 100.898) -> (191.85, 100.898)
  arc A312 (191.748, 101) -> (191.85, 100.898) centre (191.85, 101) ccw
  line L285 (191.748, 101) -> (191.748, 102.4)
  arc A313 (191.85, 102.502) -> (191.748, 102.4) centre (191.85, 102.4) ccw
  line L286 (191.85, 102.502) -> (193.35, 102.502)
  arc A314 (193.452, 102.4) -> (193.35, 102.502) centre (193.35, 102.4) ccw
  line L287 (193.452, 102.4) -> (193.452, 101)
  arc A315 (210.55, 101.4) -> (210.8, 101.65) centre (210.55, 101.65) ccw
  line L288 (210.55, 101.4) -> (209.65, 101.4)
  arc A316 (209.4, 101.65) -> (209.65, 101.4) centre (209.65, 101.65) ccw
  line L289 (209.4, 101.65) -> (209.4, 102.175)
  arc A317 (209.65, 102.425) -> (209.4, 102.175) centre (209.65, 102.175) ccw
  line L290 (209.65, 102.425) -> (210.55, 102.425)
  arc A318 (210.8, 102.175) -> (210.55, 102.425) centre (210.55, 102.175) ccw
  line L291 (210.8, 102.175) -> (210.8, 101.65)
  arc A319 (196.9, 100.798) -> (197.002, 100.9) centre (196.9, 100.9) ccw
  line L292 (196.9, 100.798) -> (195.4, 100.798)
  arc A320 (195.298, 100.9) -> (195.4, 100.798) centre (195.4, 100.9) ccw
  line L293 (195.298, 100.9) -> (195.298, 102.3)
  arc A321 (195.4, 102.402) -> (195.298, 102.3) centre (195.4, 102.3) ccw
  line L294 (195.4, 102.402) -> (196.9, 102.402)
  arc A322 (197.002, 102.3) -> (196.9, 102.402) centre (196.9, 102.3) ccw
  line L295 (197.002, 102.3) -> (197.002, 100.9)
  arc A323 (203.4, 100.798) -> (203.502, 100.9) centre (203.4, 100.9) ccw
  line L296 (203.4, 100.798) -> (201.9, 100.798)
  arc A324 (201.798, 100.9) -> (201.9, 100.798) centre (201.9, 100.9) ccw
  line L297 (201.798, 100.9) -> (201.798, 102.3)
  arc A325 (201.9, 102.402) -> (201.798, 102.3) centre (201.9, 102.3) ccw
  line L298 (201.9, 102.402) -> (203.4, 102.402)
  arc A326 (203.502, 102.3) -> (203.4, 102.402) centre (203.4, 102.3) ccw
  line L299 (203.502, 102.3) -> (203.502, 100.9)
  circle A327 centre (157.9, 100.4) radius 1.1
  circle A328 centre (176.95, 100.4) radius 1.1
  arc A329 (210.55, 99.575) -> (210.8, 99.825) centre (210.55, 99.825) ccw
  line L300 (210.55, 99.575) -> (209.65, 99.575)
  arc A330 (209.4, 99.825) -> (209.65, 99.575) centre (209.65, 99.825) ccw
  line L301 (209.4, 99.825) -> (209.4, 100.35)
  arc A331 (209.65, 100.6) -> (209.4, 100.35) centre (209.65, 100.35) ccw
  line L302 (209.65, 100.6) -> (210.55, 100.6)
  arc A332 (210.8, 100.35) -> (210.55, 100.6) centre (210.55, 100.35) ccw
  line L303 (210.8, 100.35) -> (210.8, 99.825)
  line L304 (196.9, 95.25) -> (196.9, 93.25)
  line L305 (196.9, 93.25) -> (193.7, 93.25)
  line L306 (193.7, 93.25) -> (193.7, 95.25)
  line L307 (193.7, 95.25) -> (196.9, 95.25)
  circle A333 centre (187.8, 91.15) radius 1
  circle A334 centre (202.3, 91.15) radius 1
  circle A335 centre (187.8, 88.65) radius 1
  circle A336 centre (164.94, 86.38) radius 2
  circle A337 centre (159.86, 86.38) radius 0.85
  circle A338 centre (170.02, 86.38) radius 0.85
  line L308 (188.8, 87.15) -> (188.8, 85.15)
  line L309 (188.8, 85.15) -> (186.8, 85.15)
  line L310 (186.8, 85.15) -> (186.8, 87.15)
  line L311 (186.8, 87.15) -> (188.8, 87.15)
  circle A339 centre (202.3, 86.15) radius 1
  circle A340 centre (161.13, 83.84) radius 1.1
  line L312 (196.9, 84.05) -> (196.9, 82.05)
  line L313 (196.9, 82.05) -> (193.7, 82.05)
  line L314 (193.7, 82.05) -> (193.7, 84.05)
  line L315 (193.7, 84.05) -> (196.9, 84.05)
  circle A341 centre (167.48, 81.3) radius 1.1
  circle A342 centre (122.55, 73.65) radius 2.2
  circle A343 centre (208.15, 73.55) radius 2.2
  arc A344 (161.55, 73.9205) -> (161.6442, 73.9835) centre (161.55, 74.0225) ccw
  line L316 (161.55, 73.9205) -> (160.95, 73.9205)
  arc A345 (160.848, 74.0225) -> (160.95, 73.9205) centre (160.95, 74.0225) ccw
  line L317 (160.848, 74.0225) -> (160.848, 75.3225)
  arc A346 (160.95, 75.4245) -> (160.848, 75.3225) centre (160.95, 75.3225) ccw
  line L318 (160.95, 75.4245) -> (161.55, 75.4245)
  arc A347 (161.6442, 75.3615) -> (161.55, 75.4245) centre (161.55, 75.3225) ccw
  line L319 (161.6442, 75.3615) -> (161.65, 75.3326)
  line L320 (161.65, 75.3326) -> (161.6558, 75.3615)
  arc A348 (161.75, 75.4245) -> (161.6558, 75.3615) centre (161.75, 75.3225) ccw
  line L321 (161.75, 75.4245) -> (162.35, 75.4245)
  arc A349 (162.4442, 75.3615) -> (162.35, 75.4245) centre (162.35, 75.3225) ccw
  line L322 (162.4442, 75.3615) -> (162.45, 75.3326)
  line L323 (162.45, 75.3326) -> (162.4558, 75.3615)
  arc A350 (162.55, 75.4245) -> (162.4558, 75.3615) centre (162.55, 75.3225) ccw
  line L324 (162.55, 75.4245) -> (162.85, 75.4245)
  arc A351 (162.9442, 75.3615) -> (162.85, 75.4245) centre (162.85, 75.3225) ccw
  line L325 (162.9442, 75.3615) -> (162.95, 75.3326)
  line L326 (162.95, 75.3326) -> (162.9558, 75.3615)
  arc A352 (163.05, 75.4245) -> (162.9558, 75.3615) centre (163.05, 75.3225) ccw
  line L327 (163.05, 75.4245) -> (163.35, 75.4245)
  arc A353 (163.4442, 75.3615) -> (163.35, 75.4245) centre (163.35, 75.3225) ccw
  line L328 (163.4442, 75.3615) -> (163.45, 75.3326)
  line L329 (163.45, 75.3326) -> (163.4558, 75.3615)
  arc A354 (163.55, 75.4245) -> (163.4558, 75.3615) centre (163.55, 75.3225) ccw
  line L330 (163.55, 75.4245) -> (163.85, 75.4245)
  arc A355 (163.9442, 75.3615) -> (163.85, 75.4245) centre (163.85, 75.3225) ccw
  line L331 (163.9442, 75.3615) -> (163.95, 75.3326)
  line L332 (163.95, 75.3326) -> (163.9558, 75.3615)
  arc A356 (164.05, 75.4245) -> (163.9558, 75.3615) centre (164.05, 75.3225) ccw
  line L333 (164.05, 75.4245) -> (164.35, 75.4245)
  arc A357 (164.4442, 75.3615) -> (164.35, 75.4245) centre (164.35, 75.3225) ccw
  line L334 (164.4442, 75.3615) -> (164.45, 75.3326)
  line L335 (164.45, 75.3326) -> (164.4558, 75.3615)
  arc A358 (164.55, 75.4245) -> (164.4558, 75.3615) centre (164.55, 75.3225) ccw
  line L336 (164.55, 75.4245) -> (164.85, 75.4245)
  arc A359 (164.9442, 75.3615) -> (164.85, 75.4245) centre (164.85, 75.3225) ccw
  line L337 (164.9442, 75.3615) -> (164.95, 75.3326)
  line L338 (164.95, 75.3326) -> (164.9558, 75.3615)
  arc A360 (165.05, 75.4245) -> (164.9558, 75.3615) centre (165.05, 75.3225) ccw
  line L339 (165.05, 75.4245) -> (165.35, 75.4245)
  arc A361 (165.4442, 75.3615) -> (165.35, 75.4245) centre (165.35, 75.3225) ccw
  line L340 (165.4442, 75.3615) -> (165.45, 75.3326)
  line L341 (165.45, 75.3326) -> (165.4558, 75.3615)
  arc A362 (165.55, 75.4245) -> (165.4558, 75.3615) centre (165.55, 75.3225) ccw
  line L342 (165.55, 75.4245) -> (165.85, 75.4245)
  arc A363 (165.9442, 75.3615) -> (165.85, 75.4245) centre (165.85, 75.3225) ccw
  line L343 (165.9442, 75.3615) -> (165.95, 75.3326)
  line L344 (165.95, 75.3326) -> (165.9558, 75.3615)
  arc A364 (166.05, 75.4245) -> (165.9558, 75.3615) centre (166.05, 75.3225) ccw
  line L345 (166.05, 75.4245) -> (166.35, 75.4245)
  arc A365 (166.4442, 75.3615) -> (166.35, 75.4245) centre (166.35, 75.3225) ccw
  line L346 (166.4442, 75.3615) -> (166.45, 75.3326)
  line L347 (166.45, 75.3326) -> (166.4558, 75.3615)
  arc A366 (166.55, 75.4245) -> (166.4558, 75.3615) centre (166.55, 75.3225) ccw
  line L348 (166.55, 75.4245) -> (167.15, 75.4245)
  arc A367 (167.2442, 75.3615) -> (167.15, 75.4245) centre (167.15, 75.3225) ccw
  line L349 (167.2442, 75.3615) -> (167.25, 75.3326)
  line L350 (167.25, 75.3326) -> (167.2558, 75.3615)
  arc A368 (167.35, 75.4245) -> (167.2558, 75.3615) centre (167.35, 75.3225) ccw
  line L351 (167.35, 75.4245) -> (167.95, 75.4245)
  arc A369 (168.052, 75.3225) -> (167.95, 75.4245) centre (167.95, 75.3225) ccw
  line L352 (168.052, 75.3225) -> (168.052, 74.0225)
  arc A370 (167.95, 73.9205) -> (168.052, 74.0225) centre (167.95, 74.0225) ccw
  line L353 (167.95, 73.9205) -> (167.35, 73.9205)
  arc A371 (167.2558, 73.9835) -> (167.35, 73.9205) centre (167.35, 74.0225) ccw
  line L354 (167.2558, 73.9835) -> (167.25, 74.0124)
  line L355 (167.25, 74.0124) -> (167.2442, 73.9835)
  arc A372 (167.15, 73.9205) -> (167.2442, 73.9835) centre (167.15, 74.0225) ccw
  line L356 (167.15, 73.9205) -> (166.55, 73.9205)
  arc A373 (166.4558, 73.9835) -> (166.55, 73.9205) centre (166.55, 74.0225) ccw
  line L357 (166.4558, 73.9835) -> (166.45, 74.0124)
  line L358 (166.45, 74.0124) -> (166.4442, 73.9835)
  arc A374 (166.35, 73.9205) -> (166.4442, 73.9835) centre (166.35, 74.0225) ccw
  line L359 (166.35, 73.9205) -> (166.05, 73.9205)
  arc A375 (165.9558, 73.9835) -> (166.05, 73.9205) centre (166.05, 74.0225) ccw
  line L360 (165.9558, 73.9835) -> (165.95, 74.0124)
  line L361 (165.95, 74.0124) -> (165.9442, 73.9835)
  arc A376 (165.85, 73.9205) -> (165.9442, 73.9835) centre (165.85, 74.0225) ccw
  line L362 (165.85, 73.9205) -> (165.55, 73.9205)
  arc A377 (165.4558, 73.9835) -> (165.55, 73.9205) centre (165.55, 74.0225) ccw
  line L363 (165.4558, 73.9835) -> (165.45, 74.0124)
  line L364 (165.45, 74.0124) -> (165.4442, 73.9835)
  arc A378 (165.35, 73.9205) -> (165.4442, 73.9835) centre (165.35, 74.0225) ccw
  line L365 (165.35, 73.9205) -> (165.05, 73.9205)
  arc A379 (164.9558, 73.9835) -> (165.05, 73.9205) centre (165.05, 74.0225) ccw
  line L366 (164.9558, 73.9835) -> (164.95, 74.0124)
  line L367 (164.95, 74.0124) -> (164.9442, 73.9835)
  arc A380 (164.85, 73.9205) -> (164.9442, 73.9835) centre (164.85, 74.0225) ccw
  line L368 (164.85, 73.9205) -> (164.55, 73.9205)
  arc A381 (164.4558, 73.9835) -> (164.55, 73.9205) centre (164.55, 74.0225) ccw
  line L369 (164.4558, 73.9835) -> (164.45, 74.0124)
  line L370 (164.45, 74.0124) -> (164.4442, 73.9835)
  arc A382 (164.35, 73.9205) -> (164.4442, 73.9835) centre (164.35, 74.0225) ccw
  line L371 (164.35, 73.9205) -> (164.05, 73.9205)
  arc A383 (163.9558, 73.9835) -> (164.05, 73.9205) centre (164.05, 74.0225) ccw
  line L372 (163.9558, 73.9835) -> (163.95, 74.0124)
  line L373 (163.95, 74.0124) -> (163.9442, 73.9835)
  arc A384 (163.85, 73.9205) -> (163.9442, 73.9835) centre (163.85, 74.0225) ccw
  line L374 (163.85, 73.9205) -> (163.55, 73.9205)
  arc A385 (163.4558, 73.9835) -> (163.55, 73.9205) centre (163.55, 74.0225) ccw
  line L375 (163.4558, 73.9835) -> (163.45, 74.0124)
  line L376 (163.45, 74.0124) -> (163.4442, 73.9835)
  arc A386 (163.35, 73.9205) -> (163.4442, 73.9835) centre (163.35, 74.0225) ccw
  line L377 (163.35, 73.9205) -> (163.05, 73.9205)
  arc A387 (162.9558, 73.9835) -> (163.05, 73.9205) centre (163.05, 74.0225) ccw
  line L378 (162.9558, 73.9835) -> (162.95, 74.0124)
  line L379 (162.95, 74.0124) -> (162.9442, 73.9835)
  arc A388 (162.85, 73.9205) -> (162.9442, 73.9835) centre (162.85, 74.0225) ccw
  line L380 (162.85, 73.9205) -> (162.55, 73.9205)
  arc A389 (162.4558, 73.9835) -> (162.55, 73.9205) centre (162.55, 74.0225) ccw
  line L381 (162.4558, 73.9835) -> (162.45, 74.0124)
  line L382 (162.45, 74.0124) -> (162.4442, 73.9835)
  arc A390 (162.35, 73.9205) -> (162.4442, 73.9835) centre (162.35, 74.0225) ccw
  line L383 (162.35, 73.9205) -> (161.75, 73.9205)
  arc A391 (161.6558, 73.9835) -> (161.75, 73.9205) centre (161.75, 74.0225) ccw
  line L384 (161.6558, 73.9835) -> (161.65, 74.0124)
  line L385 (161.65, 74.0124) -> (161.6442, 73.9835)
  arc A392 (174.75, 74.35) -> (175, 74.6) centre (174.75, 74.6) ccw
  line L386 (174.75, 74.35) -> (173.85, 74.35)
  arc A393 (173.6, 74.6) -> (173.85, 74.35) centre (173.85, 74.6) ccw
  line L387 (173.6, 74.6) -> (173.6, 75.125)
  arc A394 (173.85, 75.375) -> (173.6, 75.125) centre (173.85, 75.125) ccw
  line L388 (173.85, 75.375) -> (174.75, 75.375)
  arc A395 (175, 75.125) -> (174.75, 75.375) centre (174.75, 75.125) ccw
  line L389 (175, 75.125) -> (175, 74.6)
  arc A396 (157.05, 74.3) -> (157.3, 74.55) centre (157.05, 74.55) ccw
  line L390 (157.05, 74.3) -> (156.15, 74.3)
  arc A397 (155.9, 74.55) -> (156.15, 74.3) centre (156.15, 74.55) ccw
  line L391 (155.9, 74.55) -> (155.9, 75.075)
  arc A398 (156.15, 75.325) -> (155.9, 75.075) centre (156.15, 75.075) ccw
  line L392 (156.15, 75.325) -> (157.05, 75.325)
  arc A399 (157.3, 75.075) -> (157.05, 75.325) centre (157.05, 75.075) ccw
  line L393 (157.3, 75.075) -> (157.3, 74.55)
  arc A400 (160.757, 74.5575) -> (159.506, 74.619) centre (160.13, 74.5575) ccw
  line L394 (160.757, 74.5575) -> (160.754, 73.446)
  arc A401 (159.503, 73.5075) -> (160.754, 73.446) centre (160.13, 73.5075) ccw
  line L395 (159.503, 73.5075) -> (159.506, 74.619)
  arc A402 (169.397, 74.5575) -> (168.146, 74.619) centre (168.77, 74.5575) ccw
  line L396 (169.397, 74.5575) -> (169.394, 73.446)